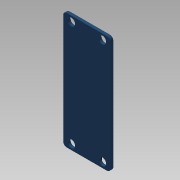
# Autodesk Inventor part: opencm
Saved by Autodesk Inventor 2014 (Build 180170000, 170)
## iProperties
Created: 2014-04-16
Part Number: opencm
Material: Générique
Document SubType Name: Modeling
Designer: Grégoire
Density: 1 g/cm^3
Appearance: Par défaut
Author: Grégoire
Autodesk Inventor part; units mm, degrees
ref_plane "YZ Plane" through (0, 0, 0) normal (1, 0, 0) x (0, 1, 0)
ref_plane "XZ Plane" through (0, 0, 0) normal (0, 1, 0) x (-1, 0, 0)
ref_plane "XY Plane" through (0, 0, 0) normal (0, 0, 1) x (1, 0, 0)
sketch "Esquisse1" plane through (0, 0, 0) normal (0, 1, 0) x (-1, 0, 0)
  line L0 (0, 0) -> (27, 0)
  line L1 (27, 0) -> (27, 66.5)
  line L2 (27, 66.5) -> (0, 66.5)
  line L3 (0, 66.5) -> (0, 0)
  line L4 (4.65, 63.35) -> (22.35, 63.35) construction
  line L5 (22.35, 63.35) -> (22.35, 3.15) construction
  line L6 (22.35, 3.15) -> (4.65, 3.15) construction
  line L7 (4.65, 3.15) -> (4.65, 63.35) construction
  line L8 (13.5, 63.35) -> (13.5, 66.5) construction
  line L9 (22.35, 33.25) -> (27, 33.25) construction
  line L10 (4.65, 33.25) -> (0, 33.25) construction
  line L11 (13.5, 3.15) -> (13.5, 0) construction
  circle A0 centre (4.65, 63.35) radius 2.15
  circle A1 centre (22.35, 63.35) radius 2.15
  circle A2 centre (4.65, 3.15) radius 2.15
  circle A3 centre (22.35, 3.15) radius 2.15
  dimension "d0" = 27
  dimension "d1" = 66.5
  dimension "d2" = 60.2
  dimension "d3" = 17.7
  dimension "d4" = 4.3
  constraints: 24 end point, 8 midpoint, 4 centre point, 4 parallel, 4 perpendicular, 3 symmetric about line, 2 horizontal, 1 coincident, 3 other
  measures "d0" distance of L0.start L0.end
  measures "d1" distance of L2.end L0.start
  measures "d2" distance of L4.end L5.end
  measures "d3" distance of L4.start L4.end
  measures "d4" diameter of A0
extrude "Extrusion1" add sketch "Esquisse1" along normal blind 1.6
fillet "Congé1" radius 2 4 edges at (0, 0.8, 0) (-27, 0.8, 0) (0, 0.8, 66.5) (-27, 0.8, 66.5)
sketch "Esquisse2" plane through (0, 1.6, 0) normal (0, 1, 0) x (1, 0, 0)
  line L0 (-2, 0) -> (-25, 0) construction
  line L1 (-18.5, 0) -> (-8.5, 0)
  line L2 (-8.5, 0) -> (-8.5, -5)
  line L3 (-8.5, -5) -> (-18.5, -5)
  line L4 (-18.5, -5) -> (-18.5, 0)
  point P0 (0, 0)
  point P1 (-13.5, 0)
  dimension "d8" = 5
  dimension "d9" = 10
  constraints: 8 end point, 2 midpoint, 2 parallel, 1 horizontal, 1 perpendicular, 1 point on line
  measures "d8" distance of L1.end L2.end
  measures "d9" distance between parallel lines of L2 L4
extrude "Extrusion2" add sketch "Esquisse2" along normal blind 2
sketch "Esquisse3" plane through (0, 1.6, 0) normal (0, 1, 0) x (1, 0, 0)
  line L0 (-6.6018, -5.2) -> (-6.6018, -9.2)
  line L1 (-6.6018, -9.2) -> (-20.6018, -9.2)
  line L2 (-20.6018, -9.2) -> (-20.6018, -5.2)
  line L3 (-18.5, -5) -> (-8.5, -5)
  line L4 (-17.7303, -5) -> (-13.5194, -5) construction
  line L5 (-13.6018, -9.2) -> (-13.6018, -29.6083) construction
  line L6 (-19.6018, -9.2) -> (-23.6018, -9.2)
  line L7 (-23.6018, -9.2) -> (-23.6018, -29.2)
  line L8 (-23.6018, -29.2) -> (-19.6018, -29.2)
  line L9 (-19.6018, -29.2) -> (-19.6018, -9.2)
  line L10 (-7.6018, -9.2) -> (-3.6018, -9.2)
  line L11 (-3.6018, -9.2) -> (-3.6018, -29.2)
  line L12 (-3.6018, -29.2) -> (-7.6018, -29.2)
  line L13 (-7.6018, -29.2) -> (-7.6018, -9.2)
  line L14 (-8.5, -5) -> (-18.5, -5)
  line L15 (-20.6018, -5.2) -> (-6.6018, -5.2)
  point P0 (0, 0)
  point P1 (-13.5, -5)
  dimension "d12" = 14
  dimension "d13" = 4
  dimension "d14" = 20
  dimension "d15" = 4
  dimension "d16" = 12
  dimension "d19" = 0.2
  constraints: 32 end point, 5 parallel, 4 symmetric about line, 2 midpoint, 2 perpendicular, 2 point on line, 1 horizontal
  measures "d12" distance between parallel lines of L0 L2
  measures "d13" distance of L0.start L0.end
  measures "d14" distance of L10.end L11.end
  measures "d15" distance of L11.end L13.start
  measures "d16" distance between parallel lines of L9 L13
  measures "d19" distance between parallel lines of L3 L15
extrude "Extrusion3" add sketch "Esquisse3" along normal blind 2
